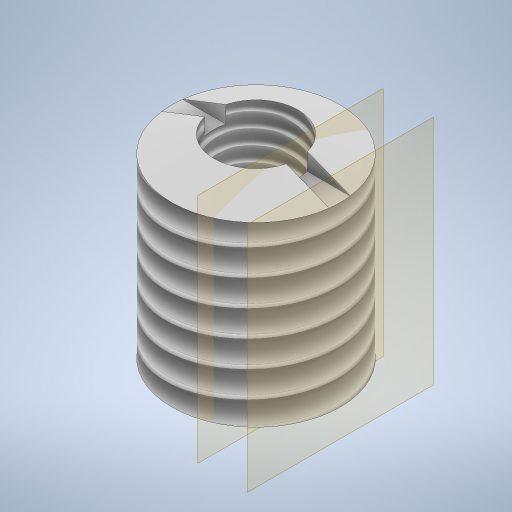
# Autodesk Inventor part: Riduttore
Saved by Autodesk Inventor 2023 (Build 270158000, 158)
## iProperties
Created: 2022-08-24
Part Number: Riduttore
Material: Generico
Document SubType Name: Modeling
Designer: matte
Density: 1 g/cm^3
Appearance: Default
Author: matte
Autodesk Inventor part; units mm, degrees
ref_plane "XZ Plane" through (0, 0, 0) normal (0, 1, 0) x (-1, 0, 0)
ref_plane "XY Plane" through (0, 0, 0) normal (0, 0, 1) x (1, 0, 0)
sketch "Schizzo1" plane through (0, 0, 0) normal (0, 1, 0) x (-1, 0, 0)
  circle A0 centre (1.635, 2.2831) radius 4
  dimension "d2" = 8
  constraints: 1 centre point
  measures "d2" diameter of A0
extrude "Estrusione1" add sketch "Schizzo1" along normal blind 10
thread "Filettatura1" size "M8x1.25" class "6g" standard "ISO Metric profile" full length
sketch "Schizzo2" plane through (-1.635, 0, 2.2831) normal (0, -1, 0) x (1, 0, 0)
  point P0 (1.635, -2.2831)
  point P1 (0, 0)
hole "Foro1" at (-1.635, 0, 2.2831) direction (0, 1, 0) diameter 4 end through all
thread "Filettatura2" size "M4x0.7" class "6H" standard "ANSI Metric M Profile" full length
chamfer "Smusso1" distance 0.8 distance2 2 2 edges at (2.365, 0, 2.2831) (2.365, 10, 2.2831) measured on face at (2.365, 9.5, 2.2831) measured on face at (2.365, 0.5, 2.2831)
ref_plane "Piano di lavoro1" through (2.365, 0, 2.2831) normal (1, 0, 0) x (0, 1, 0)
sketch "Schizzo3" plane through (2.365, 0, 2.2831) normal (1, 0, 0) x (0, 1, 0)
  line L0 (10, 2) -> (10, -2) projected
  line L1 (0, -2) -> (0, 2) projected
  line L2 (9.2, -4) -> (9.2, 4) projected
  line L3 (0.8, 4) -> (0.8, -4) projected
  line L4 (10, -0.5) -> (9.2, -0.5)
  line L5 (9.2, -0.5) -> (9.2, 0.5)
  line L6 (9.2, 0.5) -> (10, 0.5)
  line L7 (10, 0.5) -> (10, -0.5)
  line L8 (0, 0) -> (10, 0)
  line L9 (0.8, -0.5) -> (0, -0.5)
  line L10 (0, -0.5) -> (0, 0.5)
  line L11 (0, 0.5) -> (0.8, 0.5)
  line L12 (0.8, 0.5) -> (0.8, -0.5)
  point P0 (0, -2.2831)
  point P1 (0.8, 0.5)
  point P2 (0, -0.5)
  dimension "d19" = 1
  constraints: 18 end point, 5 parallel, 4 point on line, 2 horizontal, 2 midpoint, 2 perpendicular, 2 other
  measures "d19" distance between parallel lines of L4 L6
extrude "Estrusione2" cut sketch "Schizzo3" along normal through all both and the other way through all
